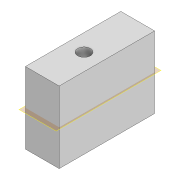
# Autodesk Inventor part: drop in nut test
Saved by Autodesk Inventor 2020 (Build 240168000, 168)
## iProperties
Created: 2019-11-26
Part Number: drop in nut test
Material: Generic
Document SubType Name: Modeling
Designer: ball
Density: 1 g/cm^3
Appearance: Default
Author: ball
Autodesk Inventor part; units mm, degrees
ref_plane "YZ Plane" through (0, 0, 0) normal (1, 0, 0) x (0, 1, 0)
ref_plane "XZ Plane" through (0, 0, 0) normal (0, 1, 0) x (-1, 0, 0)
ref_plane "XY Plane" through (0, 0, 0) normal (0, 0, 1) x (1, 0, 0)
sketch "Sketch1" plane through (0, 0, 0) normal (0, 1, 0) x (-1, 0, 0)
  line L0 (0, 0) -> (9, 0)
  line L1 (9, 0) -> (9, -25.4)
  line L2 (9, -25.4) -> (0, -25.4)
  line L3 (0, -25.4) -> (0, 0)
  dimension "d0" = 9
  dimension "d1" = 25.4
  constraints: 8 end point, 2 parallel, 1 horizontal, 1 perpendicular
  measures "d0" distance of L1.end L2.end
  measures "d1" distance of L0.end L1.end
extrude "Extrusion1" add sketch "Sketch1" along normal blind 19.05
ref_plane "Work Plane1" through (0, 9.525, 0) normal (0, 1, 0) x (1, 0, 0)
sketch "Sketch2" plane through (0, 9.525, 0) normal (0, 1, 0) x (1, 0, 0)
  circle A0 centre (-4.5, 11.1125) radius 3.45 construction
  line L0 (-9, 25.4) -> (-9, 0) projected
  line L1 (-1.05, 11.1125) -> (-2.775, 8.1247)
  line L2 (-2.775, 8.1247) -> (-9, 8.1247)
  line L3 (-9, 14.1003) -> (-2.775, 14.1003)
  line L4 (-2.775, 14.1003) -> (-1.05, 11.1125)
  line L5 (-9, 8.1247) -> (-9, 14.1003)
  point P0 (0, 0)
  dimension "d4" = 6.9
  dimension "d5" = 4.5
  constraints: 10 end point, 2 point on line, 1 coincident, 1 collinear, 1 horizontal alignment, 8 other
  measures "d5" distance from line of L0 point (-4.5, 11.113)
extrude "Extrusion2" cut sketch "Sketch2" against normal blind 4.4
sketch "Sketch3" plane through (0, 0, 0) normal (0, -1, 0) x (1, 0, 0)
  line L0 (-2.775, -8.1247) -> (-9, -8.1247) construction
  line L1 (-9, -14.1003) -> (-2.775, -14.1003) construction
  line L2 (-2.775, -14.1003) -> (-1.05, -11.1125) construction
  line L3 (-1.05, -11.1125) -> (-2.775, -8.1247) construction
  circle A0 centre (-4.5, -11.1125) radius 1.7
  line L4 (-9, -25.4) -> (-9, 0) projected
  point P0 (0, 0)
  dimension "d8" = 3.4
  dimension "d9" = 4.5
  constraints: 1 centre point
  measures "d8" diameter of A0
  measures "d9" distance from line of L4 A0.centre
extrude "Extrusion3" cut sketch "Sketch3" against normal through all
body "Solid1"
